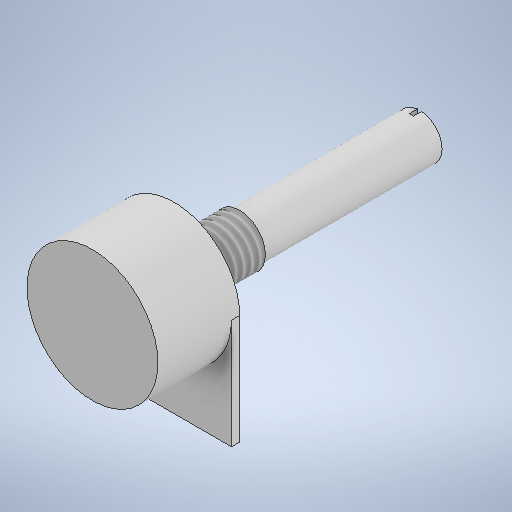
# Autodesk Inventor part: Potentiometer
Saved by Autodesk Inventor 2025.1 (Build 291241000, 241)
## iProperties
Created: 2025-05-22
Part Number: Potentiometer
Material: Generic
Document SubType Name: Modeling
Designer: Andreas' PC
Density: 1 g/cm^3
Appearance: Default
Author: Andreas' PC
Autodesk Inventor part; units mm, degrees
ref_plane "YZ Plane" through (0, 0, 0) normal (1, 0, 0) x (0, 1, 0)
ref_plane "XZ Plane" through (0, 0, 0) normal (0, 1, 0) x (-1, 0, 0)
ref_plane "XY Plane" through (0, 0, 0) normal (0, 0, 1) x (1, 0, 0)
sketch "Sketch1" plane through (0, 0, 0) normal (0, 0, 1) x (1, 0, 0)
  circle A0 centre (0, 0) radius 2.75
  line L0 (0.25, -4.8394) -> (0.25, 4.8394)
  line L1 (0.25, 4.8394) -> (-0.25, 4.8394)
  line L2 (-0.25, 4.8394) -> (-0.25, -4.8394)
  line L3 (-0.25, -4.8394) -> (0.25, -4.8394)
  line L4 (0.25, -4.8394) -> (-0.25, 4.8394) construction
  line L5 (0.25, 4.8394) -> (-0.25, -4.8394) construction
  point P0 (-0.25, 2.7386)
  point P1 (-0.25, -2.7386)
  point P2 (0.25, -2.7386)
  point P3 (0.25, 2.7386)
  dimension "d0" = 5.5
  dimension "d1" = 0.5
  constraints: 12 end point, 2 midpoint, 2 parallel, 1 centre point, 1 coincident, 1 perpendicular, 1 vertical
  measures "d0" diameter of A0
  measures "d1" distance of L1.end L0.end
extrude "Extrusion1" add sketch "Sketch1" along normal blind 30 contours A0 L0 | L0 A0 L2 | L2 A0
extrude "Extrusion2" cut sketch "Sketch1" along normal blind 1 contours L0 A0 L2
sketch "Sketch2" plane through (0, 0, 30) normal (0, 0, 1) x (1, 0, 0)
  circle A0 centre (0, 0) radius 3.15
  dimension "d6" = 6.3
  constraints: 1 centre point, 1 coincident
  measures "d6" diameter of A0
extrude "Extrusion3" add sketch "Sketch2" against normal blind 8
thread "Thread1" size "M7x1" class "6g" standard "ANSI Metric M Profile" full length
sketch "Sketch3" plane through (0, 0, 30) normal (0, 0, 1) x (1, 0, 0)
  circle A0 centre (0, 0) radius 8
  dimension "d11" = 16
  constraints: 1 centre point, 1 coincident
  measures "d11" diameter of A0
extrude "Extrusion4" add sketch "Sketch3" along normal blind 10
sketch "Sketch4" plane through (0, 0, 30) normal (0, 0, -1) x (-1, 0, 0)
  line L0 (-8, 13.3929) -> (8, 13.3929)
  line L1 (8, 13.3929) -> (8, -13.3929)
  line L2 (8, -13.3929) -> (-8, -13.3929)
  line L3 (-8, -13.3929) -> (-8, 13.3929)
  line L4 (-8, 13.3929) -> (8, -13.3929) construction
  line L5 (8, 13.3929) -> (-8, -13.3929) construction
  line L6 (8, 0) -> (-8, 0)
  circle A0 centre (0, 0) radius 8 projected
  point P0 (-5.7062, 5.6071)
  dimension "d17" = 19
  constraints: 14 end point, 4 midpoint, 2 parallel, 2 point on circle, 1 horizontal, 1 perpendicular
  measures "d17" distance from line of L2 point (-5.706, 5.607)
extrude "Extrusion5" add sketch "Sketch4" against normal blind 1 contours A0 L1 L2 L3 | L6 A0 picked at (-1.8203, -3.4339)
body "Solid1"
